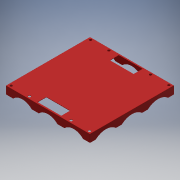
# Autodesk Inventor part: Gondola Top
Saved by Autodesk Inventor 2018 (Build 220112000, 112)
## iProperties
Created: 2018-02-08
Part Number: Gondola Top
Material: Steel, Alloy
Document SubType Name: Modeling
Designer: Joey
Density: 7.73 g/cm^3
Appearance: Smooth - Red
Author: Joey
Autodesk Inventor part; units mm, degrees
ref_plane "YZ Plane" through (0, 0, 0) normal (1, 0, 0) x (0, 1, 0)
ref_plane "XZ Plane" through (0, 0, 0) normal (0, 1, 0) x (-1, 0, 0)
ref_plane "XY Plane" through (0, 0, 0) normal (0, 0, 1) x (1, 0, 0)
sketch "Sketch1" plane through (0, 0, 0) normal (0, 0, 1) x (1, 0, 0)
  line L0 (-1076.325, 0) -> (1076.325, 0)
  line L1 (1076.325, 0) -> (1076.325, 203.2)
  line L2 (1076.325, 203.2) -> (-1076.325, 203.2)
  line L3 (-1076.325, 203.2) -> (-1076.325, 0)
  point P0 (0, 0)
  point P1 (0, 0)
  dimension "d0" = 203.2
  dimension "d1" = 2152.65
  constraints: 8 end point, 2 parallel, 1 coincident, 1 horizontal, 1 midpoint, 1 perpendicular
  measures "d0" distance of L2.end L0.start
  measures "d1" distance of L1.end L2.end
extrude "Extrusion1" add sketch "Sketch1" along normal mid plane 2152.65
shell "Shell1" thickness 9.525 removed faces 1 at (358.775, 0, 358.775)
sketch "Sketch2" plane through (0, 0, 1076.325) normal (0, 0, 1) x (1, 0, 0)
  line L0 (-1076.325, 0) -> (1076.325, 0) construction
  line L1 (1076.325, 0) -> (1076.325, 203.2) construction
  line L2 (1076.325, 203.2) -> (-1076.325, 203.2) construction
  line L3 (-1076.325, 203.2) -> (-1076.325, 0) construction
  arc A0 (-419.0259, 0) -> (-895.5722, 0) centre (-657.2991, -228.6) ccw
  arc A1 (238.2731, 0) -> (-238.2731, 0) centre (0, -228.6) ccw
  arc A2 (895.5722, 0) -> (419.0259, 0) centre (657.2991, -228.6) ccw
  line L4 (0, 0) -> (0, 101.6) construction
  line L5 (-895.5722, 0) -> (-1076.325, 0)
  line L6 (-1066.8, 193.675) -> (-1066.8, 0) construction
  line L7 (-419.0259, 0) -> (-238.2731, 0)
  line L8 (238.2731, 0) -> (419.0259, 0)
  line L9 (-1076.325, 0) -> (1076.325, 0) construction
  line L10 (895.5722, 0) -> (1076.325, 0)
  line L11 (-1076.325, 101.6) -> (1076.325, 101.6) construction
  line L12 (-895.5722, 0) -> (-419.0259, 0)
  line L13 (-238.2731, 0) -> (238.2731, 0)
  line L14 (419.0259, 0) -> (895.5722, 0)
  dimension "d5" = 330.2
  constraints: 18 end point, 7 point on circle, 5 horizontal, 3 centre point, 2 midpoint, 2 tangent, 1 collinear, 1 equal radius, 1 perpendicular, 1 vertical, 9 other
  measures "d5" radius of A1
extrude "Extrusion2" cut sketch "Sketch2" against normal through all
sketch "Sketch3" plane through (1076.325, 0, 1076.325) normal (1, 0, 0) x (0, 0, -1)
  line L0 (9.525, 0) -> (2143.125, 0) projected
  arc A0 (667.6776, 0) -> (149.6172, 0) centre (408.6474, -279.4) ccw
  arc A1 (1335.3552, 0) -> (817.2948, 0) centre (1076.325, -279.4) ccw
  arc A2 (2003.0328, 0) -> (1484.9724, 0) centre (1744.0026, -279.4) ccw
  line L1 (1076.325, 0) -> (1076.325, 101.6) construction
  line L2 (0, 203.2) -> (0, 0) construction
  line L3 (0, 101.6) -> (2152.65, 101.6)
  line L4 (2152.65, 0) -> (2152.65, 203.2) construction
  line L5 (2152.65, 0) -> (0, 0) projected
  line L6 (817.2948, 0) -> (667.6776, 0)
  line L7 (149.6172, 0) -> (0, 0)
  line L8 (1335.3552, 0) -> (1484.9724, 0)
  line L9 (2003.0328, 0) -> (2152.65, 0)
  dimension "d8" = 381
  constraints: 12 end point, 7 point on circle, 5 point on line, 4 collinear, 3 centre point, 2 midpoint, 2 tangent, 1 equal radius, 1 horizontal, 1 vertical, 3 other
  measures "d8" radius of A1
extrude "Extrusion3" cut sketch "Sketch3" against normal through all contours A0 L0 | A1 L0 | A2 L0
sketch "Sketch4" plane through (-1076.325, 203.2, 1076.325) normal (0, 1, 0) x (1, 0, 0)
  circle A0 centre (73.025, 2092.325) radius 31.75
  line L0 (9.525, 2143.125) -> (2143.125, 2143.125) projected
  line L1 (9.525, 2143.125) -> (9.525, 9.525) projected
  circle A1 centre (542.925, 2092.325) radius 31.75
  circle A2 centre (73.025, 60.325) radius 31.75
  circle A3 centre (2079.625, 2092.325) radius 31.75
  circle A4 centre (2079.625, 60.325) radius 31.75
  circle A5 centre (542.925, 60.325) radius 31.75
  circle A6 centre (1609.725, 2092.325) radius 31.75
  circle A7 centre (1609.725, 60.325) radius 31.75
  line L2 (1381.125, 34.925) -> (771.525, 34.925) construction
  line L3 (771.525, 34.925) -> (771.525, 2117.725) construction
  line L4 (771.525, 2117.725) -> (1381.125, 2117.725) construction
  line L5 (1381.125, 2117.725) -> (1381.125, 34.925) construction
  line L6 (1381.125, 34.925) -> (771.525, 2117.725) construction
  line L7 (771.525, 34.925) -> (1381.125, 2117.725) construction
  line L8 (771.525, 2117.725) -> (1381.125, 2117.725)
  line L9 (1381.125, 2117.725) -> (1381.125, 1889.125)
  line L10 (1381.125, 1889.125) -> (771.525, 1889.125)
  line L11 (771.525, 1889.125) -> (771.525, 2117.725)
  line L12 (1381.125, 34.925) -> (771.525, 34.925)
  line L13 (771.525, 34.925) -> (771.525, 263.525)
  line L14 (771.525, 263.525) -> (1381.125, 263.525)
  line L15 (1381.125, 263.525) -> (1381.125, 34.925)
  point P0 (1076.325, 1076.325)
  dimension "d11" = 63.5
  dimension "d14" = 50.8
  dimension "d15" = 63.5
  dimension "d16" = 63.5
  dimension "d17" = 533.4
  dimension "d18" = 50.8
  dimension "d21" = 2032
  dimension "d24" = 2006.6
  dimension "d29" = 2032
  dimension "d32" = 1066.8
  dimension "d37" = 609.6
  dimension "d38" = 2082.8
  dimension "d39" = 228.6
  dimension "d40" = 228.6
  constraints: 28 end point, 8 centre point, 6 parallel, 5 horizontal, 3 perpendicular, 2 midpoint, 2 point on line, 2 vertical, 12 other
  measures "d11" diameter of A0
  measures "d14" distance from line of L0 A0.centre
  measures "d15" distance from line of L1 A0.centre
  measures "d16" diameter of A1
  measures "d17" distance from line of A1.centre L1
  measures "d18" distance from line of L0 A1.centre
  measures "d21" distance of A0.centre A2.centre
  measures "d24" distance of A0.centre A3.centre
  measures "d29" distance of A1.centre A5.centre
  measures "d32" distance of A1.centre A6.centre
  measures "d37" distance of L3.end L4.end
  measures "d38" distance of L2.end L3.end
  measures "d39" distance of L8.end L9.end
  measures "d40" distance of L12.end L13.end
extrude "Extrusion4" cut sketch "Sketch4" against normal through all
fillet "Fillet1" radius 6.35 36 edges at (1076.325, 101.6, 1076.325) (0, 203.2, 1076.325) (1076.325, 203.2, 0) (-1076.325, 101.6, 1076.325) (1076.325, 101.6, -1076.325) (-1076.325, 203.2, 0) (0, 203.2, -1076.325) (-1076.325, 101.6, -1076.325) (-657.2991, 101.6, -1076.325) (0, 101.6, -1076.325) (-328.6495, 0, -1076.325) (-985.9486, 0, -1076.325) (-1076.325, 0, -1001.5164) (-1076.325, 101.6, -667.6776) (-1076.325, 0, -333.8388) (-1076.325, 101.6, 0) (-1076.325, 0, 333.8388) (-1076.325, 101.6, 667.6776) (328.6495, 0, -1076.325) (657.2991, 101.6, -1076.325) (985.9486, 0, -1076.325) (-1076.325, 0, 1001.5164) (1076.325, 0, -1001.5164) (1076.325, 101.6, -667.6776) (1076.325, 0, -333.8388) (1076.325, 101.6, 0) (1076.325, 0, 333.8388) (1076.325, 101.6, 667.6776) (1076.325, 0, 1001.5164) (985.9486, 0, 1076.325) (657.2991, 101.6, 1076.325) (328.6495, 0, 1076.325) (0, 101.6, 1076.325) (-328.6495, 0, 1076.325) (-657.2991, 101.6, 1076.325) (-985.9486, 0, 1076.325)
body "Solid1"
